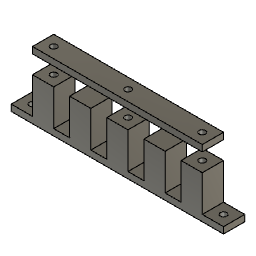
ESC Holder (Sierra) 2-6-20 (Autodesk Fusion 360 design; units mm, degrees)
Autodesk Fusion 360 part; units mm, degrees
note: some values were not read from the file. Chosen so that the rebuilt part matches the saved one: which face or edge a step refers to.
sketch "Sketch1" plane through (0, 0, 0) normal (0, 0, 1) x (1, 0, 0)
  line L0 (-8, 3.4716) -> (92, 3.4716)
  line L1 (92, 3.4716) -> (92, -6.5284)
  line L2 (92, -6.5284) -> (-8, -6.5284)
  line L3 (-8, -6.5284) -> (-8, 3.4716)
  dimension "d1" = 100
  dimension "d2" = 10
  constraint horizontal L0
  constraint vertical L1
  constraint horizontal L2
  constraint vertical L3
  measures "d1" distance of L0.start L0.end
  measures "d2" distance of L0.start L2.end
extrude "Extrude1" add sketch "Sketch1" along normal blind 17 makes body 1
sketch "Sketch5" plane through (0, 0, 17) normal (0, 0, 1) x (-1, 0, 0)
  line L0 (8, 6.5284) -> (-92, 6.5284)
  line L1 (-92, 6.5284) -> (-92, -3.4716)
  line L2 (-92, -3.4716) -> (8, -3.4716)
  line L3 (8, -3.4716) -> (8, 6.5284)
  line L4 (8, -3.4716) -> (-2, -3.4716)
  line L5 (-2, -3.4716) -> (-2, 6.5284)
  line L6 (-2, 6.5284) -> (8, 6.5284)
  line L7 (8, 6.5284) -> (8, -3.4716)
  dimension "d16" = 10
  constraint horizontal L4
  constraint vertical L5
  constraint horizontal L6
  constraint vertical L7
  constraint coincident L2.end L3.start
  measures "d16" distance of L2.end L4.end
extrude "Extrude4" cut sketch "Sketch5" against normal blind 14 contours L0 L2 L3 L4 L5 L6 L7 bodies 1
sketch "Sketch6" plane through (0, 0, 17) normal (0, 0, 1) x (-1, 0, 0)
  line L0 (-2, -3.4716) -> (-2, 6.5284)
  line L1 (-2, 6.5284) -> (-92, 6.5284)
  line L2 (-92, 6.5284) -> (-92, -3.4716)
  line L3 (-92, -3.4716) -> (-2, -3.4716)
  line L4 (-2, -3.4716) -> (-12, -3.4716)
  line L5 (-12, -3.4716) -> (-12, 6.5284)
  line L6 (-12, 6.5284) -> (-2, 6.5284)
  line L7 (-2, 6.5284) -> (-2, -3.4716)
  line L8 (-12, -3.4716) -> (-19.5, -3.4716)
  line L9 (-19.5, -3.4716) -> (-19.5, 6.5284)
  line L10 (-19.5, 6.5284) -> (-12, 6.5284)
  line L11 (-12, 6.5284) -> (-12, -3.4716)
  line L12 (-19.5, -3.4716) -> (-29.5, -3.4716)
  line L13 (-29.5, -3.4716) -> (-29.5, 6.5284)
  line L14 (-29.5, 6.5284) -> (-19.5, 6.5284)
  line L15 (-19.5, 6.5284) -> (-19.5, -3.4716)
  line L16 (-29.5, -3.4716) -> (-37, -3.4716)
  line L17 (-37, -3.4716) -> (-37, 6.5284)
  line L18 (-37, 6.5284) -> (-29.5, 6.5284)
  line L19 (-29.5, 6.5284) -> (-29.5, -3.4716)
  line L20 (-37, -3.4716) -> (-47, -3.4716)
  line L21 (-47, -3.4716) -> (-47, 6.5284)
  line L22 (-47, 6.5284) -> (-37, 6.5284)
  line L23 (-37, 6.5284) -> (-37, -3.4716)
  line L24 (-47, -3.4716) -> (-54.5, -3.4716)
  line L25 (-54.5, -3.4716) -> (-54.5, 6.5284)
  line L26 (-54.5, 6.5284) -> (-47, 6.5284)
  line L27 (-47, 6.5284) -> (-47, -3.4716)
  line L28 (-54.5, -3.4716) -> (-64.5, -3.4716)
  line L29 (-64.5, -3.4716) -> (-64.5, 6.5284)
  line L30 (-64.5, 6.5284) -> (-54.5, 6.5284)
  line L31 (-54.5, 6.5284) -> (-54.5, -3.4716)
  line L32 (-64.5, -3.4716) -> (-72, -3.4716)
  line L33 (-72, -3.4716) -> (-72, 6.5284)
  line L34 (-72, 6.5284) -> (-64.5, 6.5284)
  line L35 (-64.5, 6.5284) -> (-64.5, -3.4716)
  line L36 (-72, -3.4716) -> (-82, -3.4716)
  line L37 (-82, -3.4716) -> (-82, 6.5284)
  line L38 (-82, 6.5284) -> (-72, 6.5284)
  line L39 (-72, 6.5284) -> (-72, -3.4716)
  dimension "d19" = 10
  dimension "d20" = 7.5
  dimension "d21" = 10
  dimension "d22" = 7.5
  dimension "d23" = 7.5
  dimension "d24" = 10
  dimension "d25" = 7.5
  dimension "d26" = 10
  constraint horizontal L4
  constraint vertical L5
  constraint horizontal L6
  constraint vertical L7
  constraint coincident L1 L5.end
  constraint coincident L0.start L3.end
  constraint horizontal L8
  constraint vertical L9
  constraint horizontal L10
  constraint vertical L11
  constraint coincident L1 L9.end
  constraint horizontal L12
  constraint vertical L13
  constraint horizontal L14
  constraint vertical L15
  constraint coincident L1 L13.end
  constraint horizontal L16
  constraint vertical L17
  constraint horizontal L18
  constraint vertical L19
  constraint coincident L1 L17.end
  constraint horizontal L20
  constraint vertical L21
  constraint horizontal L22
  constraint vertical L23
  constraint midpoint L1 L21.end
  constraint horizontal L24
  constraint vertical L25
  constraint horizontal L26
  constraint vertical L27
  constraint coincident L1 L25.end
  constraint horizontal L28
  constraint vertical L29
  constraint horizontal L30
  constraint vertical L31
  constraint coincident L1 L29.end
  constraint horizontal L32
  constraint vertical L33
  constraint horizontal L34
  constraint vertical L35
  constraint coincident L1 L33.end
  constraint horizontal L36
  constraint vertical L37
  constraint horizontal L38
  constraint vertical L39
  constraint coincident L1 L37.end
  measures "d19" distance of L0.start L4.end
  measures "d20" distance of L4.end L8.end
  measures "d21" distance of L8.end L12.end
  measures "d22" distance of L12.end L16.end
  measures "d23" distance of L20.end L24.end
  measures "d24" distance of L24.end L28.end
  measures "d25" distance of L28.end L32.end
  measures "d26" distance of L32.end L36.end
extrude "Extrude5" cut sketch "Sketch6" against normal blind 14 contours L1 L3 L5 L8 L9 L10 L11 L15 | L1 L3 L13 L16 L17 L18 L19 L23 | L1 L3 L21 L24 L25 L26 L27 L31 | L1 L3 L29 L32 L33 L34 L35 L39 | L1 L2 L3 L37 bodies 1
extrude "Extrude6" add 5 faces at (5.3333, 0.1383, 17) (22.8333, 0.1383, 17) (40.3333, 0.1383, 17) (57.8333, 0.1383, 17) (78.6667, -3.195, 17) along direction (0, 0, 1) blind 3 on bodies 1 bodies 1
sketch "Sketch7" plane through (0, 0, 20) normal (0, 0, 1) x (-1, 0, 0)
  line L0 (-72, -3.4716) -> (-72, 6.5284)
  line L1 (-72, 6.5284) -> (-82, 6.5284)
  line L2 (-82, 6.5284) -> (-82, -3.4716)
  line L3 (-82, -3.4716) -> (-72, -3.4716)
  circle A0 centre (-77, 1.5284) radius 1.5
  dimension "d31" = 3
  measures "d31" diameter of A0
extrude "Extrude7" cut sketch "Sketch7" along normal blind -10 and the other way blind -17 contours A0 bodies 1
sketch "Sketch8" plane through (0, 0, 20) normal (0, 0, 1) x (-1, 0, 0)
  line L0 (-54.5, -3.4716) -> (-54.5, 6.5284)
  line L1 (-54.5, 6.5284) -> (-64.5, 6.5284)
  line L2 (-64.5, 6.5284) -> (-64.5, -3.4716)
  line L3 (-64.5, -3.4716) -> (-54.5, -3.4716)
  circle A0 centre (-42.0003, 1.5002) radius 1.5
  circle A1 centre (-6.9902, 1.5284) radius 1.5
  dimension "d34" = 3
  dimension "d35" = 3
  measures "d34" diameter of A0
  measures "d35" diameter of A1
extrude "Extrude8" cut sketch "Sketch8" against normal blind 10 contours A0 | A1 bodies 1
sketch "Sketch9" plane through (0, 0, 3) normal (0, 0, 1) x (-1, 0, 0)
  line L0 (-82, -3.4716) -> (-82, 6.5284)
  line L1 (-82, 6.5284) -> (-92, 6.5284)
  line L2 (-92, 6.5284) -> (-92, -3.4716)
  line L3 (-92, -3.4716) -> (-82, -3.4716)
  circle A0 centre (-87, 1.5) radius 1.5
  dimension "d38" = 3
  measures "d38" diameter of A0
extrude "Extrude9" cut sketch "Sketch9" against normal blind 7 contours A0 bodies 1
sketch "Sketch10" plane through (0, 0, 3) normal (0, 0, 1) x (-1, 0, 0)
  line L0 (8, 6.5284) -> (-2, 6.5284)
  line L1 (-2, 6.5284) -> (-2, -3.4716)
  line L2 (-2, -3.4716) -> (8, -3.4716)
  line L3 (8, -3.4716) -> (8, 6.5284)
  circle A0 centre (2.9957, 1.5503) radius 1.5
  dimension "d41" = 3
  measures "d41" diameter of A0
extrude "Extrude10" cut sketch "Sketch10" against normal blind 6 contours A0 bodies 1
sketch "Sketch11" plane through (0, 0, 20) normal (0, 0, 1) x (-1, 0, 0)
  circle A0 centre (-6.9902, 1.5284) radius 1.5
  line L0 (-12, 6.5284) -> (-12, -3.4716)
  line L1 (-12, -3.4716) -> (-2, -3.4716)
  line L2 (-2, -3.4716) -> (-2, 6.5284)
  line L3 (-2, 6.5284) -> (-12, 6.5284)
  line L4 (-2, -3.4716) -> (-3, -3.4716)
  line L5 (-3, -3.4716) -> (-3, -2.5)
  line L6 (-3, -2.5) -> (-2, -2.5)
  line L7 (-2, -2.5) -> (-2, -3.4716)
  constraint horizontal L4
  constraint vertical L5
  constraint horizontal L6
  constraint vertical L7
  constraint coincident L1.end L2.start
extrude "Extrude11" add sketch "Sketch11" along normal blind 5.5 contours L1 L2 L4 L5 L6 L7 bodies 1
extrude "Extrude12" add 1 faces at (2.6667, 2.8239, 25.5) along direction (0, 0, 1) blind 3 on bodies 1 bodies 1
sketch "Sketch12" plane through (0, 0, 28.5) normal (0, 0, 1) x (-1, 0, 0)
  line L0 (-2, -2.5) -> (-3, -2.5)
  line L1 (-3, -2.5) -> (-3, -3.4716)
  line L2 (-3, -3.4716) -> (-2, -3.4716)
  line L3 (-2, -3.4716) -> (-2, -2.5)
  line L4 (-2, -3.4716) -> (-82, -3.4716)
  line L5 (-82, -3.4716) -> (-82, 6.5284)
  line L6 (-82, 6.5284) -> (-2, 6.5284)
  line L7 (-2, 6.5284) -> (-2, -3.4716)
  dimension "d48" = 10
  dimension "d49" = 80
  constraint horizontal L4
  constraint vertical L5
  constraint horizontal L6
  constraint vertical L7
  constraint coincident L2.end L3.start
  measures "d48" distance of L2.end L6.end
  measures "d49" distance of L2.end L4.end
extrude "Extrude13" add sketch "Sketch12" along normal blind 3 separate body contours L0 L1 L4 L5 L6 L7 makes body 2
extrude "Extrude14" cut 1 faces at (2.6667, 2.8239, 28.5) along direction (0, 0, -1) blind 8.5 on bodies 1 bodies 1
sketch "Sketch13" plane through (0, 0, 31.5) normal (0, 0, 1) x (-1, 0, 0)
  line L0 (-2, 6.5284) -> (-82, 6.5284)
  line L1 (-82, 6.5284) -> (-82, -3.4716)
  line L2 (-82, -3.4716) -> (-3, -3.4716)
  line L3 (-3, -3.4716) -> (-3, -2.5)
  line L4 (-3, -2.5) -> (-2, -2.5)
  line L5 (-2, -2.5) -> (-2, 6.5284)
  line L6 (-3, -2.5) -> (-2.0058, -2.5)
  line L7 (-2.0058, -2.5) -> (-2.0058, -3.4716)
  line L8 (-2.0058, -3.4716) -> (-3, -3.4716)
  line L9 (-3, -3.4716) -> (-3, -2.5)
  constraint horizontal L6
  constraint vertical L7
  constraint horizontal L8
  constraint vertical L9
  constraint coincident L3.end L4.start
extrude "Extrude15" add sketch "Sketch13" against normal blind 3 contours L3 L4 L6 L7 L8 L9 bodies 2
sketch "Sketch14" plane through (0, 0, 20) normal (0, 0, 1) x (-1, 0, 0)
  circle A0 centre (-77, 1.5284) radius 1.5
  line L0 (-72, -3.4716) -> (-72, 6.5284)
  line L1 (-72, 6.5284) -> (-82, 6.5284)
  line L2 (-82, 6.5284) -> (-82, -3.4716)
  line L3 (-82, -3.4716) -> (-72, -3.4716)
  circle A1 centre (-77, 1.5284) radius 1.5
  constraint concentric A0 A1
extrude "Extrude16" cut sketch "Sketch14" along normal blind 13 contours A0 A1 bodies 2
sketch "Sketch15" plane through (0, 0, 20) normal (0, 0, 1) x (-1, 0, 0)
  circle A0 centre (-42.0003, 1.5002) radius 1.5
  line L0 (-47, 6.5284) -> (-47, -3.4716)
  line L1 (-47, -3.4716) -> (-37, -3.4716)
  line L2 (-37, -3.4716) -> (-37, 6.5284)
  line L3 (-37, 6.5284) -> (-47, 6.5284)
  circle A1 centre (-42.0003, 1.5002) radius 1.5
  dimension "d60" = 3
  constraint concentric A0 A1
  measures "d60" diameter of A1
extrude "Extrude17" cut sketch "Sketch15" along normal blind 18 contours A0 A1 bodies 2
sketch "Sketch16" plane through (0, 0, 20) normal (0, 0, 1) x (-1, 0, 0)
  line L0 (-2, -3.4716) -> (-2, 6.5284)
  line L1 (-2, 6.5284) -> (-12, 6.5284)
  line L2 (-12, 6.5284) -> (-12, -3.4716)
  line L3 (-12, -3.4716) -> (-2, -3.4716)
  circle A0 centre (-6.9902, 1.5284) radius 1.5
  circle A1 centre (-6.9902, 1.5284) radius 1.5
  dimension "d63" = 3
  constraint concentric A0 A1
  measures "d63" diameter of A1
extrude "Extrude18" cut sketch "Sketch16" along normal blind 12 contours A0 A1 bodies 2
sketch "Sketch2" plane through (0, 0, 0) normal (0, 0, 1) x (1, 0, 0)
sketch "Sketch3" plane through (0, 0, 17) normal (0, 0, 1) x (-1, 0, 0)
  line L0 (8, 6.5284) -> (-92, 6.5284)
  line L1 (-92, 6.5284) -> (-92, -3.4716)
  line L2 (-92, -3.4716) -> (8, -3.4716)
  line L3 (8, -3.4716) -> (8, 6.5284)
  line L4 (8, -3.4716) -> (3, -3.4716)
  line L5 (3, -3.4716) -> (3, 6.5284)
  line L6 (3, 6.5284) -> (8, 6.5284)
  line L7 (8, 6.5284) -> (8, -3.4716)
  dimension "d7" = 5
  constraint horizontal L4
  constraint vertical L5
  constraint horizontal L6
  constraint vertical L7
  constraint coincident L0 L5.end
  constraint coincident L2.end L3.start
  measures "d7" distance of L2.end L4.end
extrude "Extrude2" [suppressed]
sketch "Sketch4" plane through (0, 0, 17) normal (0, 0, 1) x (-1, 0, 0)
  line L0 (3, -3.4716) -> (3, 6.5284)
  line L1 (3, 6.5284) -> (-92, 6.5284)
  line L2 (-92, 6.5284) -> (-92, -3.4716)
  line L3 (-92, -3.4716) -> (3, -3.4716)
  line L4 (3, -3.4716) -> (-9, -3.4716)
  line L5 (-9, -3.4716) -> (-9, 6.5284)
  line L6 (-9, 6.5284) -> (3, 6.5284)
  line L7 (3, 6.5284) -> (3, -3.4716)
  line L8 (-9, -3.4716) -> (-16.5, -3.4716)
  line L9 (-16.5, -3.4716) -> (-16.5, 6.5284)
  line L10 (-16.5, 6.5284) -> (-9, 6.5284)
  line L11 (-9, 6.5284) -> (-9, -3.4716)
  line L12 (-16.5, -3.4716) -> (-28.5, -3.4716)
  line L13 (-28.5, -3.4716) -> (-28.5, 6.5284)
  line L14 (-28.5, 6.5284) -> (-16.5, 6.5284)
  line L15 (-16.5, 6.5284) -> (-16.5, -3.4716)
  dimension "d10" = 12
  dimension "d11" = 7.5
  dimension "d12" = 10
  dimension "d13" = 12
  constraint horizontal L4
  constraint vertical L5
  constraint horizontal L6
  constraint vertical L7
  constraint coincident L1 L5.end
  constraint coincident L0.start L3.end
  constraint horizontal L8
  constraint vertical L9
  constraint horizontal L10
  constraint vertical L11
  constraint coincident L1 L9.end
  constraint horizontal L12
  constraint vertical L13
  constraint horizontal L14
  constraint vertical L15
  measures "d10" distance of L0.start L4.end
  measures "d11" distance of L4.end L8.end
  measures "d12" distance of L8.end L9.end
  measures "d13" distance of L8.end L12.end
extrude "Extrude3" [suppressed]
